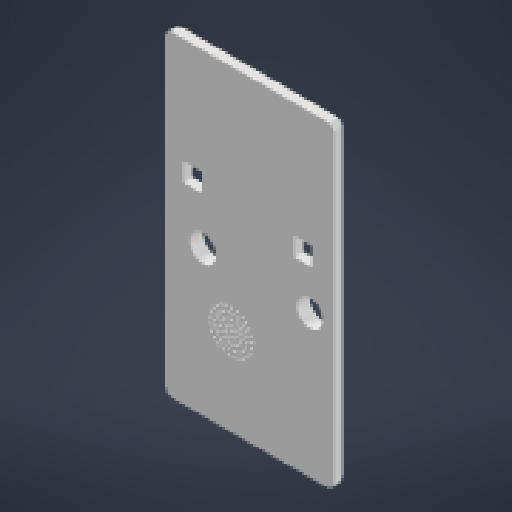
# Autodesk Inventor part: Top_Shell
Saved by Autodesk Inventor 2027 (Build 310192000, 192)
## iProperties
Created: 2026-03-03
Part Number: Top_Shell
Material: Generic
Document SubType Name: Modeling
Designer: kjedr
Density: 1 g/cm^3
Appearance: Default
Author: kjedr
Autodesk Inventor part; units mm, degrees
ref_plane "YZ Plane" through (0, 0, 0) normal (1, 0, 0) x (0, 1, 0)
ref_plane "XZ Plane" through (0, 0, 0) normal (0, 1, 0) x (-1, 0, 0)
ref_plane "XY Plane" through (0, 0, 0) normal (0, 0, 1) x (1, 0, 0)
sketch "Sketch1" plane through (0, 0, 0) normal (0, 0, 1) x (1, 0, 0)
  line L0 (0, 0) -> (80.8355, 0)
  line L1 (80.8355, 0) -> (80.8355, 152.4)
  line L2 (80.8355, 152.4) -> (0, 152.4)
  line L3 (0, 152.4) -> (0, 0)
  dimension "d0" = 80.8355
  dimension "d1" = 152.4
  constraints: 8 end point, 3 perpendicular, 1 horizontal
  measures "d0" distance of L2.end L1.end
  measures "d1" distance of L1.end L0.end
extrude "Extrusion1" add sketch "Sketch1" along normal blind 6.35
fillet "Fillet1" radius 3.175 8 edges at (80.8355, 152.4, 3.175) (0, 152.4, 3.175) (40.4178, 152.4, 0) (80.8355, 76.2, 0) (40.4177, 0, 0) (0, 76.2, 0) (0, 0, 3.175) (80.8355, 0, 3.175)
sketch "Sketch8" plane through (0, 0, 0) normal (0, 0, -1) x (-1, 0, 0)
  circle A0 centre (-31.7043, 41.9898) radius 12.7 construction
  circle A1 centre (-31.7043, 41.9898) radius 10.16 construction
  circle A2 centre (-31.7043, 41.9898) radius 7.62 construction
  circle A3 centre (-31.7043, 41.9898) radius 5.08 construction
  circle A4 centre (-31.7043, 41.9898) radius 2.54 construction
  line L0 (-80.8355, 149.225) -> (-80.8355, 3.175) projected
  line L1 (-77.6605, 0) -> (-3.175, 0) projected
  point P0 (0, 0)
  point P1 (-29.2552, 42.6633)
  point P2 (-36.6993, 41.0645)
  point P3 (-24.1328, 42.8482)
  point P4 (-22.1292, 45.3874)
  point P5 (-23.275, 47.6618)
  point P6 (-24.9504, 49.5799)
  point P7 (-27.0501, 51.0211)
  point P8 (-29.4424, 51.8948)
  point P9 (-31.9767, 52.1461)
  point P10 (-34.4939, 51.7593)
  point P11 (-36.8359, 50.7586)
  point P12 (-38.8554, 49.2069)
  point P13 (-40.4255, 47.2018)
  point P14 (-41.4477, 44.8691)
  point P15 (-41.8577, 42.3556)
  point P16 (-41.6297, 39.819)
  point P17 (-40.778, 37.4189)
  point P18 (-39.3562, 35.3059)
  point P19 (-37.4536, 33.613)
  point P20 (-35.1898, 32.4463)
  point P21 (-32.7069, 31.8794)
  point P22 (-30.161, 31.9477)
  point P23 (-27.7122, 32.6469)
  point P24 (-25.5141, 33.9332)
  point P25 (-23.705, 35.7258)
  point P26 (-22.3985, 37.9119)
  point P27 (-21.6768, 40.3543)
  point P28 (-21.5851, 42.8994)
  point P29 (-24.7686, 45.1459)
  point P30 (-26.0834, 47.1347)
  point P31 (-27.9483, 48.6198)
  point P32 (-30.1809, 49.4559)
  point P33 (-32.5627, 49.5613)
  point P34 (-34.8604, 48.9254)
  point P35 (-36.8492, 47.6107)
  point P36 (-38.3343, 45.7457)
  point P37 (-39.1704, 43.5131)
  point P38 (-39.2758, 41.1313)
  point P39 (-38.6399, 38.8336)
  point P40 (-37.3252, 36.8449)
  point P41 (-35.4602, 35.3597)
  point P42 (-33.2276, 34.5236)
  point P43 (-30.8458, 34.4183)
  point P44 (-28.5481, 35.0541)
  point P45 (-26.5594, 36.3689)
  point P46 (-25.0742, 38.2338)
  point P47 (-24.2381, 40.4664)
  point P48 (-35.8911, 39.1129)
  point P49 (-34.359, 37.6586)
  point P50 (-32.3679, 36.9533)
  point P51 (-30.262, 37.1188)
  point P52 (-28.4055, 38.1266)
  point P53 (-27.1194, 39.8023)
  point P54 (-26.626, 41.8562)
  point P55 (-27.0107, 43.9333)
  point P56 (-28.207, 45.6743)
  point P57 (-30.008, 46.7782)
  point P58 (-32.1023, 47.0541)
  point P59 (-34.1278, 46.4544)
  point P60 (-35.7342, 45.0827)
  point P61 (-36.6438, 43.1762)
  point P62 (-30.4487, 44.1978)
  point P63 (-32.3778, 44.4388)
  point P64 (-33.9123, 43.2453)
  point P65 (-34.1533, 41.3163)
  point P66 (-32.9598, 39.7818)
  point P67 (-31.0308, 39.5407)
  point P68 (-29.4963, 40.7343)
  dimension "d39" = 20.32
  dimension "d40" = 15.24
  dimension "d41" = 10.16
  dimension "d42" = 5.08
  dimension "d38" = 25.4
  dimension "d45" = 360
  dimension "d49" = 360
  dimension "d53" = 360
  dimension "d57" = 360
  constraints: 5 coincident, 1 centre point, 84 other
  measures "d38" diameter of A0
hole "Hole1" at (31.7043, 41.9898, 0) at (29.2552, 42.6633, 0) at (36.6993, 41.0645, 0) at (24.1328, 42.8482, 0) at (22.1292, 45.3874, 0) at (23.275, 47.6618, 0) at (24.9504, 49.5799, 0) at (27.0501, 51.0211, 0) at (29.4424, 51.8948, 0) at (31.9767, 52.1461, 0) at (34.4939, 51.7593, 0) at (36.8359, 50.7586, 0) at (38.8554, 49.2069, 0) at (40.4255, 47.2018, 0) at (41.4477, 44.8691, 0) at (41.8577, 42.3556, 0) at (41.6297, 39.819, 0) at (40.778, 37.4189, 0) at (39.3562, 35.3059, 0) at (37.4536, 33.613, 0) at (35.1898, 32.4463, 0) at (32.7069, 31.8794, 0) at (30.161, 31.9477, 0) at (27.7122, 32.6469, 0) at (25.5141, 33.9332, 0) at (23.705, 35.7258, 0) at (22.3985, 37.9119, 0) at (21.6768, 40.3543, 0) at (21.5851, 42.8994, 0) at (24.7686, 45.1459, 0) at (26.0834, 47.1347, 0) at (27.9483, 48.6198, 0) at (30.1809, 49.4559, 0) at (32.5627, 49.5613, 0) at (34.8604, 48.9254, 0) at (36.8492, 47.6107, 0) at (38.3343, 45.7457, 0) at (39.1704, 43.5131, 0) at (39.2758, 41.1313, 0) at (38.6399, 38.8336, 0) at (37.3252, 36.8449, 0) at (35.4602, 35.3597, 0) at (33.2276, 34.5236, 0) at (30.8458, 34.4183, 0) at (28.5481, 35.0541, 0) at (26.5594, 36.3689, 0) at (25.0742, 38.2338, 0) at (24.2381, 40.4664, 0) at (35.8911, 39.1129, 0) at (34.359, 37.6586, 0) direction (0, 0, 1) diameter 1.27 end through all and at (32.3679, 36.9533, 0) (30.262, 37.1188, 0) (28.4055, 38.1266, 0) (27.1194, 39.8023, 0) (26.626, 41.8562, 0) (27.0107, 43.9333, 0) (28.207, 45.6743, 0) (30.008, 46.7782, 0) (32.1023, 47.0541, 0) (34.1278, 46.4544, 0) (35.7342, 45.0827, 0) (36.6438, 43.1762, 0) (30.4487, 44.1978, 0) (32.3778, 44.4388, 0) (33.9123, 43.2453, 0) (34.1533, 41.3163, 0) (32.9598, 39.7818, 0) (31.0308, 39.5407, 0) (29.4963, 40.7343, 0)
sketch "Sketch12" plane through (0, 0, 0) normal (0, 0, -1) x (-1, 0, 0)
  point P0 (0, 0)
sketch "Sketch14" plane through (0, 0, 0) normal (0, 0, -1) x (-1, 0, 0)
  line L0 (-75.6868, 90.81) -> (-5.1488, 90.81) construction
  line L1 (-5.1488, 90.81) -> (-5.1488, 6.81) construction
  line L2 (-5.1488, 6.81) -> (-75.6868, 6.81) construction
  line L3 (-75.6868, 6.81) -> (-75.6868, 90.81) construction
  circle A0 centre (-75.2472, 83.516) radius 1.6
  circle A1 centre (-13.6268, 83.516) radius 1.6
  circle A2 centre (-75.2472, 22.81) radius 1.6
  circle A3 centre (-13.6268, 22.81) radius 1.6
  line L4 (-77.6605, 149.225) -> (-3.175, 149.225) projected
  line L5 (-77.0255, 3.81) -> (-3.81, 3.81) projected
  point P0 (0, 0)
  point P1 (-40.4178, 90.81)
  point P2 (-40.4178, 125.7733)
  point P3 (-69.4004, 68.5651)
  point P4 (-18.0721, 69.8455)
  point P5 (-40.4178, 6.81)
  point P6 (-40.4178, 149.225)
  dimension "d90" = 3.2
  constraints: 8 end point, 4 centre point, 4 vertical alignment, 3 equal radius, 3 midpoint, 2 horizontal alignment, 2 parallel, 1 horizontal, 1 perpendicular
  measures "d90" diameter of A0
hole "Hole4" at (69.4004, 68.5651, 0) at (18.0721, 69.8455, 0) direction (0, 0, 1) diameter 12.7 end through all
sketch "Sketch21" plane through (0, 0, 0) normal (0, 0, -1) x (-1, 0, 0)
  line L0 (-72.5632, 98.9087) -> (-59.8632, 98.9087)
  line L1 (-59.8632, 98.9087) -> (-59.8632, 86.2087)
  line L2 (-59.8632, 86.2087) -> (-72.5632, 86.2087)
  line L3 (-72.5632, 86.2087) -> (-72.5632, 98.9087)
  line L4 (-72.5632, 98.9087) -> (-59.8632, 86.2087) construction
  line L5 (-59.8632, 98.9087) -> (-72.5632, 86.2087) construction
  line L6 (-19.4778, 103.3537) -> (-6.7778, 103.3537)
  line L7 (-6.7778, 103.3537) -> (-6.7778, 90.6537)
  line L8 (-6.7778, 90.6537) -> (-19.4778, 90.6537)
  line L9 (-19.4778, 90.6537) -> (-19.4778, 103.3537)
  line L10 (-19.4778, 103.3537) -> (-6.7778, 90.6537) construction
  line L11 (-6.7778, 103.3537) -> (-19.4778, 90.6537) construction
  line L12 (-70.6582, 97.0037) -> (-61.7682, 97.0037)
  line L13 (-61.7682, 97.0037) -> (-61.7682, 88.1137)
  line L14 (-61.7682, 88.1137) -> (-70.6582, 88.1137)
  line L15 (-70.6582, 88.1137) -> (-70.6582, 97.0037)
  line L16 (-70.6582, 97.0037) -> (-61.7682, 88.1137) construction
  line L17 (-61.7682, 97.0037) -> (-70.6582, 88.1137) construction
  line L18 (-77.6605, 0) -> (-3.175, 0) projected
  circle A0 centre (-31.7043, 41.9898) radius 0.635 projected
  line L19 (-17.5728, 101.4487) -> (-8.6828, 101.4487)
  line L20 (-8.6828, 101.4487) -> (-8.6828, 92.5587)
  line L21 (-8.6828, 92.5587) -> (-17.5728, 92.5587)
  line L22 (-17.5728, 92.5587) -> (-17.5728, 101.4487)
  line L23 (-17.5728, 101.4487) -> (-8.6828, 92.5587) construction
  line L24 (-8.6828, 101.4487) -> (-17.5728, 92.5587) construction
  line L25 (0, 3.175) -> (0, 149.225) projected
  line L26 (-3.175, 152.4) -> (-77.6605, 152.4) projected
  point P0 (0, 0)
  point P1 (-66.2132, 92.5587)
  point P2 (-13.1278, 97.0037)
  dimension "d143" = 12.7
  dimension "d144" = 12.7
  dimension "d145" = 12.7
  dimension "d146" = 12.7
  dimension "d147" = 8.89
  dimension "d150" = 8.89
  dimension "d151" = 8.89
  constraints: 48 end point, 8 midpoint, 8 parallel, 4 horizontal, 4 perpendicular, 1 point on line
  measures "d143" distance of L1.end L2.end
  measures "d144" distance of L0.end L1.end
  measures "d145" distance of L7.end L8.end
  measures "d146" distance of L6.end L7.end
  measures "d147" distance of L13.end L14.end
  measures "d150" distance of L20.end L21.end
  measures "d151" distance of L19.end L20.end
extrude "Extrusion10" cut sketch "Sketch21" against normal blind 6.35 contours L12 L13 L14 L15 | L19 L20 L21 L22
extrude "Extrusion11" cut sketch "Sketch21" against normal blind 1.905 contours L0 L1 L2 L3 | L6 L7 L8 L9 | L19 L20 L21 L22
body "Solid1"
